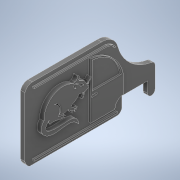
# Autodesk Inventor part: right_panel
Saved by Autodesk Inventor 2022 (Build 260153000, 153)
## iProperties
Created: 2021-06-17
Part Number: right_panel
Material: Plastic, Opaque Black
Document SubType Name: Modeling
Designer: kevin
Density: 0.952 g/cm^3
Appearance: Smooth - Black
Author: kevin
Autodesk Inventor part; units mm, degrees
ref_plane "YZ Plane" through (0, 0, 0) normal (1, 0, 0) x (0, 1, 0)
ref_plane "XZ Plane" through (0, 0, 0) normal (0, 1, 0) x (-1, 0, 0)
ref_plane "XY Plane" through (0, 0, 0) normal (0, 0, 1) x (1, 0, 0)
sketch "outline" plane through (0, 0, 0) normal (1, 0, 0) x (0, 1, 0)
  line L0 (0, 88.9038) -> (127, 88.9038) construction
  line L1 (127, 88.9038) -> (127, -88.8962) construction
  line L2 (127, -88.8962) -> (0, -88.8962) construction
  line L3 (0, -88.8962) -> (0, 88.9038) construction
  line L4 (0, 88.9038) -> (127, -88.8962) construction
  line L5 (127, 88.9038) -> (0, -88.8962) construction
  line L6 (-6.35, -82.5462) -> (38.1, -82.5462)
  line L7 (38.1, -82.5462) -> (38.1, -44.4462)
  line L8 (38.1, -44.4462) -> (-6.35, -44.4462)
  line L9 (-6.35, -44.4462) -> (-6.35, -82.5462)
  line L10 (4.9871, -50.7075) -> (22.0805, -50.7075) construction
  line L11 (22.0805, -50.7075) -> (22.0805, -80.6209) construction
  line L12 (22.0805, -80.6209) -> (4.9871, -80.6209) construction
  line L13 (4.9871, -80.6209) -> (4.9871, -50.7075) construction
  line L14 (179.262, 0.0038) -> (-38.2255, 0.0038) construction
  line L15 (0, 150.8125) -> (0, -173.0375) construction
  point P0 (63.5, 0.0038)
  point P1 (63.5, 0.0038)
  dimension "d0" = 177.8
  dimension "d1" = 127
  dimension "d2" = 38.1
  dimension "d3" = 44.45
  dimension "d4" = 6.35
  dimension "d5" = 6.35
  constraints: 24 end point, 4 horizontal, 4 parallel, 3 midpoint, 2 perpendicular, 2 vertical, 1 collinear, 1 point on line, 2 other
  measures "d0" distance of L0.end L1.end
  measures "d1" distance of L1.end L2.end
  measures "d2" distance of L8.end L6.start
  measures "d3" distance of L6.start L6.end
  measures "d4" distance between parallel lines of L6 L2
  measures "d5" distance between parallel lines of L9 L15
sketch "Sketch2" plane through (0, 0, 0) normal (1, 0, 0) x (0, 1, 0)
  line L0 (16.1492, -36.7509) -> (16.1492, 92.075)
  line L1 (25.5684, 98.5943) -> (113.7408, 98.5943)
  line L2 (121.8722, 87.4339) -> (121.8722, -14.7243)
  line L3 (38.1007, -44.45) -> (38.1007, -82.55)
  line L4 (38.1007, -44.45) -> (12.7007, -44.45)
  line L5 (38.1007, -82.55) -> (17.4632, -82.55)
  arc A0 (121.8722, 87.4339) -> (113.7408, 98.5943) centre (110.1475, 87.4339) ccw
  line L6 (31.7507, -44.45) -> (31.7507, 88.9) construction
  line L7 (25.4007, -44.45) -> (25.4007, 88.9) construction
  circle A1 centre (56.4395, 60.4012) radius 2.3813
  line L8 (0, -88.9) -> (117.475, -88.9) construction
  arc A2 (22.225, -82.55) -> (22.225, -93.6625) centre (22.225, -88.1063) ccw
  line L9 (22.225, -93.6625) -> (52.3875, -93.6625)
  arc A3 (104.2778, -38.5424) -> (58.7375, -88.9) centre (120.3654, -98.8617) ccw
  arc A4 (104.2778, -38.5424) -> (121.8722, -14.7243) centre (98.1639, -15.6185) ccw
  arc A5 (16.1492, -36.7509) -> (25.4007, -44.45) centre (23.7736, -36.9971) ccw
  arc A6 (25.5684, 98.5943) -> (16.1492, 92.075) centre (28.7116, 83.9887) ccw
  arc A7 (52.3875, -93.6625) -> (58.7375, -88.9) centre (53.0922, -87.9875) ccw
  point P0 (0, 0)
  point P1 (22.1466, -44.45)
  dimension "d6" = 6.35
  dimension "d7" = 6.35
  dimension "d8" = 4.7625
  dimension "d9" = 24.6888
  dimension "d10" = 149.3012
  constraints: 20 end point, 14 point on circle, 8 centre point, 8 horizontal, 6 vertical, 4 tangent, 2 midpoint, 2 point on line
  measures "d6" distance between parallel lines of L6 L3
  measures "d7" distance between parallel lines of L7 L6
  measures "d8" diameter of A1
  measures "d9" distance from line of L6 A1.centre
  measures "d10" distance from line of A1.centre L8
extrude "main right panel" add sketch "Sketch2" along normal blind 6.35 contours L0 A6 L1 A0 L2 A4 A3 A7 L9 A2 L5 L3 L4 A5
sketch "rat icon raw" plane through (6.35, 0, 0) normal (1, 0, 0) x (0, 0, -1)
  line L0 (-53.1267, 106.3625) -> (-10.9673, 106.3625) construction
  line L1 (-10.9673, 106.3625) -> (-10.9673, 68.2625) construction
  line L2 (-10.9673, 68.2625) -> (-53.1267, 68.2625) construction
  line L3 (-53.1267, 68.2625) -> (-53.1267, 106.3625) construction
  line L4 (-80.9625, 106.3625) -> (-14.2875, 106.3625) construction
  line L5 (-80.9625, 68.2625) -> (-14.2875, 68.2625) construction
  point P0 (0, 0)
  constraints: 4 end point, 4 horizontal, 2 collinear, 2 other
sketch "detail lines" plane through (6.35, 0, 0) normal (1, 0, 0) x (0, 0, -1)
  line L0 (41.275, 68.2625) -> (-1.5875, 68.2625)
  line L1 (-1.5875, 68.2625) -> (-1.5875, 107.95)
  arc A0 (41.275, 68.2625) -> (-1.5875, 107.95) centre (-4.3356, 61.9925) ccw
  line L2 (-4.1415, 110.938) -> (-4.1415, 28.575)
  line L3 (-4.1415, 28.575) -> (31.75, 28.575)
  arc A1 (44.45, 66.675) -> (-4.1415, 110.938) centre (-10.0865, 55.6085) ccw
  line L4 (44.45, 66.675) -> (44.45, 41.275)
  arc A2 (44.45, 41.275) -> (31.75, 28.575) centre (44.45, 28.575) ccw
  line L5 (-1.5875, 61.9925) -> (4.7625, 61.9925) construction
  line L6 (-1.5875, 60.4851) -> (4.7625, 60.4851)
  line L7 (4.7625, 63.5) -> (-1.5875, 63.5)
  arc A3 (-1.5875, 63.5) -> (-1.5875, 60.4851) centre (-1.5875, 61.9925) ccw
  arc A4 (4.7625, 60.4851) -> (4.7625, 63.5) centre (4.7625, 61.9925) ccw
  line L8 (35.4697, 23.6503) -> (-87.3125, 23.6503)
  line L9 (-87.4339, 115.8875) -> (19.8438, 115.8875)
  arc A5 (33.3375, 107.95) -> (19.8438, 115.8875) centre (17.1097, 95.8012) ccw
  line L10 (-87.4339, 115.8875) -> (-87.4339, 114.3)
  line L11 (-87.4339, 114.3) -> (18.8487, 114.3)
  arc A6 (31.75, 107.1391) -> (18.8487, 114.3) centre (18.8487, 99.0979) ccw
  line L12 (31.75, 107.1391) -> (33.3375, 107.95)
  line L13 (-87.3125, 23.6503) -> (-87.3125, 21.5255)
  line L14 (-87.3125, 21.5255) -> (35.4697, 21.5255)
  line L15 (35.4697, 21.5255) -> (35.4697, 23.6503)
  point P0 (0, 0)
  point P1 (1.5875, 61.9925)
  constraints: 34 end point, 14 point on circle, 7 centre point, 5 perpendicular, 5 tangent, 4 horizontal, 4 vertical, 1 midpoint, 1 parallel
extrude "car details extrusion" add sketch "detail lines" along normal blind 2.54
sketch "rat sketch" plane through (6.35, 0, 0) normal (1, 0, 0) x (0, 0, -1)
  spline S0 degree 4 poles (-25.1113, 40.168) (-30.3286, 62.8002) (-40.2895, 47.0939) (-91.8199, 45.4722) (-69.0311, 66.7314) knots 0 0 0 0 0 1 1 1 1 1
  spline S1 degree 4 poles (-25.1113, 40.168) (-44.8827, 65.0652) (-62.3129, 21.5895) (-100.0449, 58.8688) (-70.6074, 74.0707) knots 0 0 0 0 0 1 1 1 1 1
  arc A0 (-69.0311, 66.7314) -> (-67.585, 61.8172) centre (-67.0769, 64.6366) ccw
  arc A1 (-49.2116, 58.7947) -> (-67.585, 61.8172) centre (-65.5506, 16.8269) ccw
  line L0 (-49.2116, 58.7947) -> (-50.6913, 60.6928)
  line L1 (-50.6913, 60.6928) -> (-46.1556, 58.7947)
  line L2 (-46.1556, 58.7947) -> (-48.7906, 62.1746)
  line L3 (-48.7906, 62.1746) -> (-44.7522, 60.4847)
  line L4 (-44.7522, 60.4847) -> (-47.0983, 63.4939)
  arc A2 (-55.3235, 64.9029) -> (-47.0983, 63.4939) centre (-49.5283, 74.0213) ccw
  arc A3 (-55.3235, 64.9029) -> (-61.4396, 83.2385) centre (-66.0407, 71.5159) ccw
  arc A4 (-55.3235, 64.9029) -> (-61.4396, 83.2385) centre (-62.9686, 72.5406) ccw
  arc A5 (-54.0945, 66.3736) -> (-40.9879, 66.7314) centre (-47.8743, 78.7553) ccw
  arc A6 (-40.9879, 66.7314) -> (-36.1311, 63.3712) centre (-37.5728, 66.4775) ccw
  arc A7 (-33.4791, 95.4623) -> (-76.7213, 69.5945) centre (-48.4257, 71.3709) ccw
  arc A8 (-36.1311, 63.3712) -> (-34.9888, 58.791) centre (16.1312, 73.9736) ccw
  line L5 (-34.9888, 58.791) -> (-34.9888, 62.1708)
  line L6 (-34.9888, 62.1708) -> (-32.1742, 61.0684)
  line L7 (-32.1742, 61.0684) -> (-30.8802, 58.791)
  line L8 (-30.8802, 58.791) -> (-31.2041, 61.6196)
  line L9 (-31.2041, 61.6196) -> (-32.1742, 62.8915)
  line L10 (-32.1742, 62.8915) -> (-30.6857, 62.8915)
  line L11 (-30.6857, 62.8915) -> (-29.0402, 60.4346)
  line L12 (-29.0402, 60.4346) -> (-29.0402, 62.3815)
  line L13 (-29.0402, 62.3815) -> (-29.9306, 63.7109)
  line L14 (-29.9306, 63.7109) -> (-27.2529, 62.8915)
  line L15 (-27.2529, 62.8915) -> (-28.2579, 64.392)
  arc A9 (-28.2579, 64.392) -> (-33.7777, 64.8449) centre (-31.6378, 57.0631) ccw
  arc A10 (-34.8841, 70.1283) -> (-33.7777, 64.8449) centre (-32.3651, 67.8983) ccw
  arc A11 (-34.8841, 70.1283) -> (-23.8004, 78.7218) centre (-46.3737, 96.3917) ccw
  arc A12 (-23.8004, 78.7218) -> (-15.5306, 77.1344) centre (-17.1285, 91.1448) ccw
  line L16 (-15.5306, 77.1344) -> (-13.4262, 78.7736)
  arc A13 (-13.4262, 78.7736) -> (-12.5498, 83.2524) centre (-12.73, 80.9625) ccw
  line L17 (-12.5498, 83.2524) -> (-17.1338, 91.6691)
  line L18 (-17.1338, 91.6691) -> (-22.5552, 93.9422)
  arc A14 (-24.7828, 98.5157) -> (-22.5552, 93.9422) centre (-22.0776, 97.0041) ccw
  arc A15 (-24.7828, 98.5157) -> (-27.2583, 102.3227) centre (-27.0229, 99.7674) ccw
  arc A16 (-30.6895, 96.6707) -> (-27.2583, 102.3227) centre (-32.5957, 101.6955) ccw
  arc A17 (-30.6895, 96.6707) -> (-33.4791, 95.4623) centre (-19.0133, 65.8926) ccw
  arc A18 (-17.8515, 86.2944) -> (-24.7683, 89.3504) centre (-22.6941, 84.6895) ccw
  arc A19 (-24.7558, 89.356) -> (-17.8515, 86.2944) centre (-19.1737, 92.6286) ccw
  arc A20 (-32.5957, 93.9422) -> (-29.4854, 87.2366) centre (-28.196, 91.9088) ccw
  arc A21 (-25.7638, 91.6691) -> (-32.5957, 93.9422) centre (-30.7455, 88.0996) ccw
  arc A22 (-26.408, 91.1448) -> (-31.0346, 92.4063) centre (-29.6597, 88.3339) ccw
  arc A23 (-31.0346, 92.4063) -> (-29.0402, 87.4607) centre (-25.1113, 91.9201) ccw
  line L19 (-29.0402, 87.4607) -> (-29.4854, 87.2366)
  line L20 (-26.408, 91.1448) -> (-25.7638, 91.6691)
  line L21 (-19.1737, 77.1927) -> (-22.6941, 72.5406)
  line L22 (-22.6941, 72.5406) -> (-22.6941, 71.6578)
  line L23 (-22.6941, 71.6578) -> (-18.6565, 77.1266)
  line L24 (-20.5712, 69.8924) -> (-17.5596, 76.9468)
  line L25 (-20.5712, 69.8924) -> (-20.5712, 70.2775)
  line L26 (-20.5712, 70.2775) -> (-17.8411, 77.0616)
  line L27 (-17.5935, 76.8675) -> (-18.3698, 71.0148)
  line L28 (-18.3698, 71.0148) -> (-18.1898, 70.2775)
  line L29 (-18.1898, 70.2775) -> (-17.2434, 76.8211)
  line L30 (-17.2434, 76.8211) -> (-17.2434, 77.0441)
  line L31 (-12.5498, 83.2524) -> (-9.4887, 86.2944)
  line L32 (-9.4887, 86.2944) -> (-11.9194, 84.6895)
  line L33 (-11.9194, 84.6895) -> (-6.9637, 91.1448)
  line L34 (-6.9637, 91.1448) -> (-12.5498, 85.492)
  line L35 (-12.5498, 85.492) -> (-11.3289, 88.6625)
  line L36 (-11.3289, 88.6625) -> (-13.0786, 85.5794)
  line L37 (-13.0786, 85.5794) -> (-13.5578, 85.1032)
  point P0 (0, 0)
  point P1 (-32.5957, 51.1893)
  point P2 (-50.6956, 51.4518)
  point P3 (-71.9355, 54.0894)
  point P4 (-46.3737, 47.5886)
  point P5 (-67.5516, 46.5674)
  point P6 (-79.7754, 55.7354)
  point P7 (-18.6565, 77.1266)
  constraints: 76 end point, 56 point on circle, 24 centre point, 6 parallel, 5 vertical, 3 point on line, 2 tangent, 1 coincident, 1 horizontal, 1 perpendicular, 14 other
extrude "rat extrusion" add sketch "rat sketch" along normal blind 6.35 contours S1 A7 A17 A16 A15 A14 L18 L17 A13 L16 A12 A11 A10 A9 L15 L14 L13 L12 L11 L10 L9 L8 L7 L6 L5 A8 A6 A5 A4 A3 A2 L4 L3 L2 L1 L0 A1 A0 S0 | L37 L36 L35 L34 L33 L32 L31 L17 | L30 L29 L28 L27 L24 L25 L26 A12 | L23 L22 L21 A12
body "Solid1"
